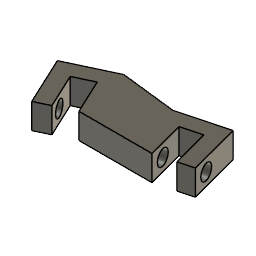
slide_v2 (Autodesk Fusion 360 design; units mm, degrees)
Autodesk Fusion 360 part; units mm, degrees
sketch "Sketch1" plane through (0, 0, 0) normal (0, 0, 1) x (1, 0, 0)
  line L0 (-14.0117, 5.1007) -> (-10.388, 6.7944)
  line L1 (-6.577, -1.3589) -> (-10.388, 6.7944)
  line L2 (-10.2007, -3.0527) -> (-14.0117, 5.1007)
  line L3 (-6.577, -1.3589) -> (-10.2007, -3.0527)
  line L4 (5.2862, 7.2485) -> (9.1521, 8.2757)
  line L5 (11.4632, -0.4225) -> (9.1521, 8.2757)
  line L6 (7.5974, -1.4497) -> (5.2862, 7.2485)
  line L7 (11.4632, -0.4225) -> (7.5974, -1.4497)
  line L8 (-6.577, -1.3589) -> (-7.2122, 0)
  line L9 (7.5974, -1.4497) -> (7.2122, 0)
  line L10 (7.2122, 0) -> (-7.2122, 0)
  line L11 (-7.2122, 0) -> (-10.8359, -1.6938) construction
  line L12 (7.2122, 0) -> (11.078, 1.0272) construction
  line L13 (-10.8359, -1.6938) -> (-13.5536, -2.9641)
  line L14 (-13.5536, -2.9641) -> (-17.9998, 6.5481)
  line L15 (-17.9998, 6.5481) -> (-9.0742, 10.72)
  line L16 (11.078, 1.0272) -> (13.9774, 1.7975)
  line L17 (13.9774, 1.7975) -> (11.2811, 11.9454)
  line L18 (11.2811, 11.9454) -> (1.8852, 9.4489)
  line L19 (1.8852, 9.4489) -> (-9.0742, 10.72)
  line L20 (10.3077, 3.9266) -> (13.2071, 4.6969)
  line L21 (6.4418, 2.8994) -> (3.5424, 2.129)
  line L22 (-12.1062, 1.024) -> (-8.4825, 2.7178)
  line L23 (-8.4825, 2.7178) -> (-5.7647, 3.9881)
  line L24 (-5.7647, 3.9881) -> (-14.824, -0.2463)
  line L25 (3.5424, 2.129) -> (13.2071, 4.6969)
  dimension "d1" = 4
  dimension "d2" = 9
  dimension "d3" = 9
  dimension "d4" = 4
  dimension "d5" = 9
  dimension "d6" = 9
  dimension "d7" = 1.5
  dimension "d8" = 1.5
  dimension "d9" = 14.4243
  dimension "d10" = 64.948
  dimension "d11" = 104.88
  dimension "d12" = 3
  dimension "d13" = 3
  dimension "d14" = 3
  dimension "d15" = 3
  dimension "d16" = 3
  dimension "d17" = 3
  constraint perpendicular L5 L7
  constraint perpendicular L6 L7
  constraint coincident L4.end L5
  constraint perpendicular L4 L5
  constraint perpendicular L2 L3
  constraint perpendicular L1 L3
  constraint perpendicular L3 L8
  constraint perpendicular L7 L9
  constraint coincident L2 L11.end
  constraint perpendicular L2 L11
  constraint coincident L5 L12.end
  constraint perpendicular L5 L12
  constraint coincident origin L10
  constraint midpoint origin L10
  constraint horizontal L10
  constraint perpendicular L2 L13
  constraint perpendicular L0 L14
  constraint perpendicular L14 L15
  constraint perpendicular L5 L16
  constraint perpendicular L16 L17
  constraint perpendicular L17 L18
  constraint midpoint L5 L20.start
  constraint midpoint L6 L21.start
  constraint coincident L17 L20.end
  constraint perpendicular L17 L20
  constraint perpendicular L6 L21
  constraint midpoint L2 L22.start
  constraint midpoint L1 L22.end
  constraint perpendicular L1 L23
  constraint coincident L14 L24.end
  constraint perpendicular L14 L24
  measures "d1" distance of L6.start L5.start
  measures "d2" distance of L4.end L5.start
  measures "d3" distance of L4.start L6.start
  measures "d4" distance of L1.start L2.start
  measures "d5" distance of L0.start L2.start
  measures "d6" distance of L1.start L0.end
  measures "d7" distance of L1.start L8.end
  measures "d8" distance of L6.start L9.end
  measures "d9" horizontal distance of L8.end L9.end
  measures "d10" angle of L1 L10
  measures "d11" angle of L9 L10
  measures "d12" distance of L11.end L13.end
  measures "d13" distance of L12.end L16.end
  measures "d14" distance of L0 L15
  measures "d15" distance of L4 L18
  measures "d16" distance of L21.start L21.end
  measures "d17" distance of L22.end L23.end
extrude "Extrude1" add sketch "Sketch1" along normal blind 3 and the other way blind 2 contours L0 L1 L2 L4 L5 L6 L10 L14 L15 L17 L18 L19 L20 L24 L25 | L2 L13 L14 L24 | L5 L16 L17 L20 L25
sketch "Sketch2" plane through (-9.5427, -4.4604, 0) normal (0.905923, 0.423442, 0) x (-0.423442, 0.905923, 0)
  line L0 (10.5539, -2) -> (10.5539, 3)
  line L1 (10.5539, 3) -> (3.0539, 3)
  line L2 (3.0539, 3) -> (3.0539, -2)
  line L3 (3.0539, -2) -> (10.5539, -2)
  line L4 (10.5539, 0.5) -> (6.0539, 0.5) construction
  circle A0 centre (6.0539, 0.5) radius 1.5
  dimension "d22" = 4.5
  dimension "d23" = 3
  constraint midpoint L0 L4.start
  constraint perpendicular L0 L4
  constraint coincident L4.end A0.centre
  measures "d22" distance of L4.start L4.end
  measures "d23" diameter of A0
extrude "Extrude2" cut sketch "Sketch2" along normal blind 7 and the other way blind 7.5 contours A0
sketch "Sketch3" plane through (10.6025, 2.8171, 0) normal (-0.966467, -0.256791, 0) x (0.256791, -0.966467, 0)
  line L0 (1.852, -2) -> (1.852, 3)
  line L1 (1.852, 3) -> (-5.648, 3)
  line L2 (-5.648, 3) -> (-5.648, -2)
  line L3 (-5.648, -2) -> (1.852, -2)
  circle A0 centre (-1.148, 0.5) radius 1.5
  line L4 (-1.148, 0.5) -> (-5.648, 0.5)
  dimension "d28" = 3
  dimension "d31" = 4.5
  constraint coincident A0.centre L4.start
  constraint midpoint L2 L4.end
  constraint perpendicular L2 L4
  measures "d28" diameter of A0
  measures "d31" distance of A0.centre L4.end
extrude "Extrude3" cut sketch "Sketch3" against normal blind 9 contours A0
extrude "Extrude4" cut sketch "Sketch3" along normal blind 7 contours A0
